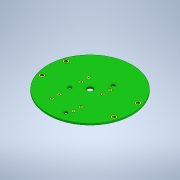
# Autodesk Inventor part: CC-PCB
Saved by Autodesk Inventor 2020 (Build 240168000, 168)
## iProperties
Created: 2019-07-03
Part Number: CC-PCB
Material: Generic
Document SubType Name: Modeling
Designer: andwh
Density: 1 g/cm^3
Appearance: Dark Green
Author: andwh
Autodesk Inventor part; units mm, degrees
ref_plane "YZ Plane" through (0, 0, 0) normal (1, 0, 0) x (0, 1, 0)
ref_plane "XZ Plane" through (0, 0, 0) normal (0, 1, 0) x (-1, 0, 0)
ref_plane "XY Plane" through (0, 0, 0) normal (0, 0, 1) x (1, 0, 0)
sketch "Sketch1" plane through (0, 0, 0) normal (0, 1, 0) x (-1, 0, 0)
  circle A0 centre (0, 0) radius 44.45
  circle A1 centre (38.1, -12.7) radius 1.5
  circle A2 centre (-38.1, -12.7) radius 1.5
  circle A3 centre (38.1, 12.7) radius 1.5
  circle A4 centre (-38.1, 12.7) radius 1.5
  circle A5 centre (-11.43, -2.12) radius 0.65
  circle A6 centre (-11.43, -9.88) radius 0.65
  circle A7 centre (-9, -15.5) radius 1.775
  line L0 (11.43, -9.88) -> (-11.43, -9.88) construction
  circle A8 centre (11.43, -2.12) radius 0.65
  circle A9 centre (11.43, -9.88) radius 0.65
  arc A10 (-17.5, -5) -> (17.5, -5) centre (0, -5) ccw construction
  circle A11 centre (11.43, 21.12) radius 0.65
  circle A12 centre (-11.43, 28.88) radius 0.65
  circle A13 centre (11.43, 28.88) radius 0.65
  circle A14 centre (-9, 34.5) radius 1.775
  arc A15 (17.5, 24) -> (-17.5, 24) centre (0, 24) ccw construction
  circle A16 centre (-11.43, 21.12) radius 0.65
  circle A17 centre (12, 9.5) radius 1.775
  line L1 (17.5, -5) -> (17.5, 24) construction
  line L2 (11.43, -2.12) -> (11.43, 21.12) construction
  line L3 (0, -5) -> (0, 24) construction
  line L4 (-17.5, 24) -> (-17.5, -5) construction
  line L5 (-9, -15.5) -> (-9, 34.5) construction
  circle A18 centre (0, 0) radius 3.05
  point P0 (0, -22.5)
  point P1 (0, -9.88)
  point P2 (0, 41.5)
  point P3 (-9, 9.5)
  point P4 (11.43, 9.5)
  point P5 (0, 9.5)
  dimension "d0" = 88.9
  dimension "d1" = 3
  dimension "d2" = 76.2
  dimension "d3" = 25.4
  dimension "d4" = 17.5
  dimension "d6" = 6.1
  dimension "d7" = 64
  dimension "d8" = 3.55
  dimension "d9" = 12
  dimension "d10" = 50
  dimension "d11" = 9
  dimension "d12" = 22.86
  dimension "d13" = 7.76
  dimension "d14" = 7.76
  dimension "d15" = 23.24
  dimension "d16" = 1.3
  dimension "d17" = 12.7
  dimension "d18" = 38.1
  dimension "d38" = 9.5
  constraints: 19 centre point, 14 end point, 12 coincident, 12 equal radius, 9 vertical alignment, 8 horizontal alignment, 6 point on circle, 4 midpoint, 4 tangent, 3 vertical, 1 horizontal, 1 parallel, 1 point on line
  measures "d0" diameter of A0
  measures "d1" diameter of A1
  measures "d2" distance of A1.centre A2.centre
  measures "d3" distance of A1.centre A3.centre
  measures "d4" radius of A10
  measures "d6" diameter of A18
  measures "d7" distance of point (0, 41.5) point (0, -22.5)
  measures "d8" diameter of A17
  measures "d9" distance from line of L3 A17.centre
  measures "d10" distance of L5.start L5.end
  measures "d11" distance between parallel lines of L3 L5
  measures "d12" distance of L0.start L0.end
  measures "d13" distance of L2.start L0.start
  measures "d14" distance of point (11.43, 28.88) L2.end
  measures "d15" distance of L2.start L2.end
  measures "d16" diameter of A9
  measures "d17" vertical distance of A0.centre A1.centre
  measures "d18" horizontal distance of A1.centre A0.centre
  measures "d38" distance of point (0, 0) point (0, 9.5)
extrude "Extrusion1" add sketch "Sketch1" along normal blind 1.6
sketch "Sketch2" plane through (0, 1.6, 0) normal (0, 1, 0) x (1, 0, 0)
  circle A0 centre (0, 0) radius 44.45 construction
  circle A1 centre (-11.43, -28.88) radius 0.65 projected
  circle A2 centre (-11.43, 9.88) radius 0.65 projected
  circle A3 centre (11.43, 2.12) radius 0.65 projected
  circle A4 centre (9, -34.5) radius 1.775 construction
  circle A5 centre (11.43, 9.88) radius 0.65 projected
  circle A6 centre (38.1, -12.7) radius 1.5 projected
  circle A7 centre (-11.43, -21.12) radius 0.65 projected
  circle A8 centre (11.43, -28.88) radius 0.65 projected
  circle A9 centre (9, 15.5) radius 1.775 construction
  circle A10 centre (0, 0) radius 3.05 construction
  circle A11 centre (-11.43, 2.12) radius 0.65 projected
  circle A12 centre (-38.1, 12.7) radius 1.5 projected
  circle A13 centre (-38.1, -12.7) radius 1.5 projected
  circle A14 centre (11.43, -21.12) radius 0.65 projected
  circle A15 centre (-12, -9.5) radius 1.775 construction
  circle A16 centre (38.1, 12.7) radius 1.5 projected
  circle A17 centre (-38.1, 12.7) radius 2.5
  circle A18 centre (-38.1, -12.7) radius 2.5
  circle A19 centre (38.1, -12.7) radius 2.5
  circle A20 centre (38.1, 12.7) radius 2.5
  circle A21 centre (-11.43, -21.12) radius 1.65
  circle A22 centre (-11.43, -28.88) radius 1.65
  circle A23 centre (11.43, -21.12) radius 1.65
  circle A24 centre (11.43, -28.88) radius 1.65
  circle A25 centre (11.43, 2.12) radius 1.65
  circle A26 centre (11.43, 9.88) radius 1.65
  circle A27 centre (-11.43, 9.88) radius 1.65
  circle A28 centre (-11.43, 2.12) radius 1.65
  dimension "d24" = 1
  dimension "d25" = 1
  dimension "d26" = 1
  dimension "d27" = 1
  dimension "d28" = 1
  dimension "d29" = 1
  dimension "d30" = 1
  dimension "d31" = 1
  dimension "d32" = 1
  dimension "d33" = 1
  dimension "d34" = 1
  dimension "d35" = 1
  constraints: 12 centre point
  measures "d24" radial gap between concentric circles of A12 A17
  measures "d25" radial gap between concentric circles of A13 A18
  measures "d26" radial gap between concentric circles of A6 A19
  measures "d27" radial gap between concentric circles of A16 A20
  measures "d28" radial gap between concentric circles of A7 A21
  measures "d29" radial gap between concentric circles of A1 A22
  measures "d30" radial gap between concentric circles of A14 A23
  measures "d31" radial gap between concentric circles of A8 A24
  measures "d32" radial gap between concentric circles of A3 A25
  measures "d33" radial gap between concentric circles of A5 A26
  measures "d34" radial gap between concentric circles of A2 A27
  measures "d35" radial gap between concentric circles of A11 A28
extrude "Extrusion2" cut sketch "Sketch2" against normal blind 0.01 contours A1 | A2 | A3 | A5 | A6 | A7 | A8 | A11 | A12 | A13 | A14 | A16 | A17 | A18 | A19 | A20 | A21 | A22 | A23 | A24 | A25 | A26 | A27 | A28
equation "\"d2\" = 2 * d19"
equation "\"d3\" = 2 * d20"
equation "\"d14\" = d13"
equation "\"d19\" = 38.1"
equation "\"d20\" = 12.7"
body "Solid1"
